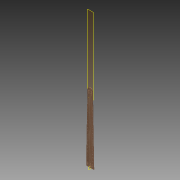
# Autodesk Inventor part: octoBotoStemSectC_v01
Saved by Autodesk Inventor 2013 (Build 170138000, 138)
## iProperties
Created: 2014-08-26
Part Number: octoBotoStemSectC_v01
Material: Wood (Birch)
Document SubType Name: Modeling
Designer: Nano
Density: 0.55 g/cm^3
Mass: 53.7405 g
Surface Area: 713.877 cm^2
Volume: 97.71 cm^3
Author: Nano
Autodesk Inventor part; units mm, degrees
ref_plane "YZ Plane" through (0, 0, 0) normal (1, 0, 0) x (0, 1, 0)
ref_plane "XZ Plane" through (0, 0, 0) normal (0, 1, 0) x (-1, 0, 0)
ref_plane "XY Plane" through (0, 0, 0) normal (0, 0, 1) x (1, 0, 0)
ref_plane "Work Plane1" through (0, 0, 0) normal (0, 0, 1) x (1, 0, 0)
sketch "Sketch1" plane through (0, 0, 0) normal (0, 0, 1) x (1, 0, 0)
  circle A0 centre (8.9214, -256.756) radius 1.651 projected
  circle A1 centre (-3.7786, -256.756) radius 1.651 projected
  circle A2 centre (-16.4786, -256.756) radius 1.651 projected
  circle A3 centre (8.9214, -263.106) radius 1.651 projected
  circle A4 centre (-3.7786, -263.106) radius 1.651 projected
  circle A5 centre (-16.4786, -263.106) radius 1.651 projected
  circle A6 centre (8.9214, -269.456) radius 1.651 projected
  circle A7 centre (-3.7786, -269.456) radius 1.651 projected
  circle A8 centre (-16.4786, -269.456) radius 1.651 projected
  circle A9 centre (8.9214, -275.806) radius 1.651 projected
  circle A10 centre (-3.7786, -275.806) radius 1.651 projected
  circle A11 centre (-16.4786, -275.806) radius 1.651 projected
  circle A12 centre (8.9214, -282.156) radius 1.651 projected
  circle A13 centre (-3.7786, -282.156) radius 1.651 projected
  circle A14 centre (-16.4786, -282.156) radius 1.651 projected
  circle A15 centre (-10.1286, -282.156) radius 1.651 projected
  circle A16 centre (2.5714, -282.156) radius 1.651 projected
  circle A17 centre (15.2714, -282.156) radius 1.651 projected
  circle A18 centre (-10.1286, -275.806) radius 1.651 projected
  circle A19 centre (2.5714, -275.806) radius 1.651 projected
  circle A20 centre (15.2714, -275.806) radius 1.651 projected
  circle A21 centre (-10.1286, -269.456) radius 1.651 projected
  circle A22 centre (2.5714, -269.456) radius 1.651 projected
  circle A23 centre (15.2714, -269.456) radius 1.651 projected
  circle A24 centre (-10.1286, -263.106) radius 1.651 projected
  circle A25 centre (2.5714, -263.106) radius 1.651 projected
  circle A26 centre (15.2714, -263.106) radius 1.651 projected
  circle A27 centre (-10.1286, -256.756) radius 1.651 projected
  circle A28 centre (2.5714, -256.756) radius 1.651 projected
  circle A29 centre (15.2714, -256.756) radius 1.651 projected
  circle A30 centre (0, 268.3019) radius 1.651 projected
  circle A31 centre (0, 274.6519) radius 1.651 projected
  circle A32 centre (0, 281.0019) radius 1.651 projected
  circle A33 centre (0, 287.3519) radius 1.651 projected
  circle A34 centre (0, 293.7019) radius 1.651 projected
  circle A35 centre (-6.35, 268.3019) radius 1.651 projected
  circle A36 centre (-6.35, 274.6519) radius 1.651 projected
  circle A37 centre (-6.35, 281.0019) radius 1.651 projected
  circle A38 centre (-6.35, 287.3519) radius 1.651 projected
  circle A39 centre (-6.35, 293.7019) radius 1.651 projected
  circle A40 centre (6.35, 268.3019) radius 1.651 projected
  circle A41 centre (6.35, 274.6519) radius 1.651 projected
  circle A42 centre (6.35, 281.0019) radius 1.651 projected
  circle A43 centre (6.35, 287.3519) radius 1.651 projected
  circle A44 centre (6.35, 293.7019) radius 1.651 projected
  arc A45 (12.0569, 296.4968) -> (-12.0569, 296.4968) centre (0, 296.336) ccw projected
  line L0 (-12.0569, 296.4968) -> (-22.8877, -285.2719) projected
  line L1 (-19.7132, -288.506) -> (19.7132, -288.506) projected
  line L2 (22.8877, -285.2719) -> (12.0569, 296.4968) projected
  arc A46 (22.3491, -256.3399) -> (-22.3491, -256.3399) centre (0, -256.756) ccw
  line L3 (-22.3491, -256.3399) -> (-32.1074, -780.5031)
  line L4 (-33.0532, -831.3031) -> (-32.8358, -831.3031)
  line L5 (33.0532, -831.3031) -> (32.1074, -780.5031)
  line L6 (-21.7296, -234.4031) -> (21.8639, -234.4031) construction
  line L7 (0.0672, -822.6817) -> (0.0672, -739.4136) construction
  arc A47 (19.7132, -288.506) -> (22.8877, -285.2719) centre (19.7132, -285.331) ccw projected
  arc A48 (-22.8877, -285.2719) -> (-19.7132, -288.506) centre (-19.7132, -285.331) ccw projected
  ellipse E0 centre (6.5498, 251.1604) end of major axis (6.5498, 245.486) minor radius 1.5875 projected
  ellipse E1 centre (7.0226, 225.7648) end of major axis (7.0226, 220.0904) minor radius 1.5875 projected
  ellipse E2 centre (7.4954, 200.3692) end of major axis (7.4954, 194.6948) minor radius 1.5875 projected
  ellipse E3 centre (7.9682, 174.9736) end of major axis (7.9682, 169.2992) minor radius 1.5875 projected
  ellipse E4 centre (8.441, 149.578) end of major axis (8.441, 143.9036) minor radius 1.5875 projected
  ellipse E5 centre (8.9138, 124.1824) end of major axis (8.9138, 118.508) minor radius 1.5875 projected
  ellipse E6 centre (9.3865, 98.7868) end of major axis (9.3865, 93.1124) minor radius 1.5875 projected
  ellipse E7 centre (9.8593, 73.3912) end of major axis (9.8593, 67.7168) minor radius 1.5875 projected
  ellipse E8 centre (10.3321, 47.9956) end of major axis (10.3321, 42.3212) minor radius 1.5875 projected
  ellipse E9 centre (10.8049, 22.6) end of major axis (10.8049, 16.9256) minor radius 1.5875 projected
  ellipse E10 centre (11.2777, -2.7956) end of major axis (11.2777, -8.47) minor radius 1.5875 projected
  ellipse E11 centre (11.7505, -28.1912) end of major axis (11.7505, -33.8656) minor radius 1.5875 projected
  ellipse E12 centre (12.2233, -53.5868) end of major axis (12.2233, -59.2611) minor radius 1.5875 projected
  ellipse E13 centre (12.6961, -78.9824) end of major axis (12.6961, -84.6567) minor radius 1.5875 projected
  ellipse E14 centre (13.1689, -104.378) end of major axis (13.1689, -110.0523) minor radius 1.5875 projected
  ellipse E15 centre (13.6417, -129.7736) end of major axis (13.6417, -135.4479) minor radius 1.5875 projected
  ellipse E16 centre (14.1145, -155.1692) end of major axis (14.1145, -160.8435) minor radius 1.5875 projected
  ellipse E17 centre (14.5872, -180.5648) end of major axis (14.5872, -186.2391) minor radius 1.5875 projected
  ellipse E18 centre (15.06, -205.9604) end of major axis (15.06, -211.6347) minor radius 1.5875 projected
  ellipse E19 centre (15.5328, -231.356) end of major axis (15.5328, -237.0303) minor radius 1.5875 projected
  ellipse E20 centre (-6.5498, 251.1604) end of major axis (-6.5498, 245.486) minor radius 1.5875 projected
  ellipse E21 centre (-7.0226, 225.7648) end of major axis (-7.0226, 220.0904) minor radius 1.5875 projected
  ellipse E22 centre (-7.4954, 200.3692) end of major axis (-7.4954, 194.6948) minor radius 1.5875 projected
  ellipse E23 centre (-7.9682, 174.9736) end of major axis (-7.9682, 169.2992) minor radius 1.5875 projected
  ellipse E24 centre (-8.441, 149.578) end of major axis (-8.441, 143.9036) minor radius 1.5875 projected
  ellipse E25 centre (-8.9138, 124.1824) end of major axis (-8.9138, 118.508) minor radius 1.5875 projected
  ellipse E26 centre (-9.3865, 98.7868) end of major axis (-9.3865, 93.1124) minor radius 1.5875 projected
  ellipse E27 centre (-9.8593, 73.3912) end of major axis (-9.8593, 67.7168) minor radius 1.5875 projected
  ellipse E28 centre (-10.3321, 47.9956) end of major axis (-10.3321, 42.3212) minor radius 1.5875 projected
  ellipse E29 centre (-10.8049, 22.6) end of major axis (-10.8049, 16.9256) minor radius 1.5875 projected
  ellipse E30 centre (-11.2777, -2.7956) end of major axis (-11.2777, -8.47) minor radius 1.5875 projected
  ellipse E31 centre (-11.7505, -28.1912) end of major axis (-11.7505, -33.8656) minor radius 1.5875 projected
  ellipse E32 centre (-12.2233, -53.5868) end of major axis (-12.2233, -59.2611) minor radius 1.5875 projected
  ellipse E33 centre (-12.6961, -78.9824) end of major axis (-12.6961, -84.6567) minor radius 1.5875 projected
  ellipse E34 centre (-13.1689, -104.378) end of major axis (-13.1689, -110.0523) minor radius 1.5875 projected
  ellipse E35 centre (-13.6417, -129.7736) end of major axis (-13.6417, -135.4479) minor radius 1.5875 projected
  ellipse E36 centre (-14.1145, -155.1692) end of major axis (-14.1145, -160.8435) minor radius 1.5875 projected
  ellipse E37 centre (-14.5872, -180.5648) end of major axis (-14.5872, -186.2391) minor radius 1.5875 projected
  ellipse E38 centre (-15.06, -205.9604) end of major axis (-15.06, -211.6347) minor radius 1.5875 projected
  ellipse E39 centre (-15.5328, -231.356) end of major axis (-15.5328, -237.0303) minor radius 1.5875 projected
  arc A49 (-25.3598, -780.5031) -> (-32.8358, -831.3031) centre (1413.9333, -1018.2666) ccw
  line L8 (25.3598, -780.5031) -> (-25.3598, -780.5031)
  arc A50 (3.175, -1364.5328) -> (32.8358, -831.3031) centre (-1413.9333, -1018.2666) ccw
  line L9 (-38.9952, -780.5031) -> (-32.1074, -780.5031)
  line L10 (32.1074, -780.5031) -> (22.3491, -256.3399)
  line L11 (-32.1074, -780.5031) -> (-33.0532, -831.3031)
  line L12 (25.3598, -780.5031) -> (32.1074, -780.5031)
  line L13 (-25.3598, -780.5031) -> (25.3598, -780.5031)
  line L14 (-32.1074, -780.5031) -> (-25.3598, -780.5031)
  line L15 (32.1074, -780.5031) -> (38.5839, -780.5031)
  arc A51 (32.8358, -831.3031) -> (25.3598, -780.5031) centre (-1413.9333, -1018.2666) ccw
  line L16 (-32.8358, -831.3031) -> (32.8358, -831.3031)
  line L17 (32.8358, -831.3031) -> (33.0532, -831.3031)
  arc A52 (-32.8358, -831.3031) -> (-3.175, -1364.5328) centre (1413.9333, -1018.2666) ccw
  point P0 (0, 0)
  dimension "d0" = 596.9
  dimension "d12" = 0
  constraints: 30 end point, 10 point on circle, 5 centre point, 5 horizontal, 4 collinear, 4 tangent, 2 point on line, 1 vertical, 50 other
  measures "d0" distance between parallel lines of L4 L6
  measures "d12" vertical distance of A2.centre A46.centre
extrude "Extrusion1" add sketch "Sketch1" along normal blind 3.175 contours L2 A47 L1 A48 L0 A46 | L10 L12 L8 L14 L3 A48 L1 A47 | A51 L16 A49 L8
sketch "Sketch2" plane through (0, 0, 3.175) normal (0, 0, 1) x (1, 0, 0)
  line L0 (-22.3491, -256.3399) -> (-32.1074, -780.5031) projected
  ellipse E0 centre (-25.2834, -755.1031) end of major axis (-25.2834, -748.7531) minor radius 1.5875
  line L1 (-32.1074, -780.5031) -> (-25.3598, -780.5031) projected
  point P0 (-33.0532, -831.3031)
  point P1 (0, 0)
  dimension "d15" = 6.35
  dimension "d17" = 1.5875
  dimension "d19" = 6.35
  dimension "d25" = 25.4
  constraints: 2 other
  measures "d19" distance from line of L0 point (-25.283, -755.103)
  measures "d25" distance from line of L1 point (-25.283, -755.103)
extrude "Extrusion2" cut sketch "Sketch2" against normal through all
ref_plane "Work Plane2" through (0, -831.3031, 3.175) normal (1, 0, 0) x (0, 1, 0)
pattern_linear "Rectangular Pattern1" count 19 spacing 25.4 along (0.0186138, 0.9998267, 0) of "Extrusion2"
mirror "Mirror1" about plane through (0, -831.3031, 3.175) normal (1, 0, 0) of "Extrusion2", "Rectangular Pattern1"
fillet "Fillet1" radius 6.35 2 edges at (32.1074, -780.5031, 1.5875) (-32.1074, -780.5031, 1.5875)
body "Solid1"
